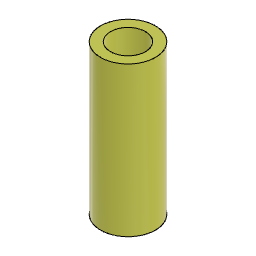
Spacer (Autodesk Fusion 360 design; units mm, degrees)
Autodesk Fusion 360 part; units mm, degrees
sketch "Skizze1" plane through (0, 0, 0) normal (0, 0, 1) x (1, 0, 0)
  circle A0 centre (0, 0) radius 1.75
  circle A1 centre (0, 0) radius 2.75
  dimension "d63" = 3.5
  dimension "d64" = 5.5
  constraint coincident A0.centre A1.centre
  constraint concentric A0 A1
  measures "d63" diameter of A0
  measures "d64" diameter of A1
extrude "Extrusion1" add sketch "Skizze1" along normal blind 15
